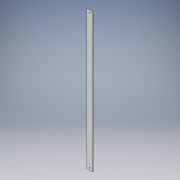
# Autodesk Inventor part: Strutural Integrity Bar
Saved by Autodesk Inventor 2018 (Build 220112000, 112)
## iProperties
Created: 2019-01-10
Part Number: Strutural Integrity Bar
Material: Generic
Document SubType Name: Modeling
Designer: maste
Density: 1 g/cm^3
Appearance: Default
Author: maste
Autodesk Inventor part; units mm, degrees
ref_plane "YZ Plane" through (0, 0, 0) normal (1, 0, 0) x (0, 1, 0)
ref_plane "XZ Plane" through (0, 0, 0) normal (0, 1, 0) x (-1, 0, 0)
ref_plane "XY Plane" through (0, 0, 0) normal (0, 0, 1) x (1, 0, 0)
sketch "Sketch1" plane through (0, 0, 0) normal (0, 0, 1) x (1, 0, 0)
  line L0 (0, 0) -> (25.4, 0)
  line L1 (25.4, 0) -> (25.4, 635)
  line L2 (25.4, 635) -> (0, 635)
  line L3 (0, 635) -> (0, 0)
  line L4 (12.7, 0) -> (12.7, 10.3251) construction
  circle A0 centre (12.7, 10.3251) radius 2.5797
  line L5 (12.7, 635) -> (12.7, 624.6749) construction
  circle A1 centre (12.7, 624.6749) radius 2.5797
  dimension "d0" = 25.4
  dimension "d1" = 635
  dimension "d2" = 10.3251
  dimension "d3" = 5.1594
  dimension "d4" = 10.3251
  constraints: 12 end point, 2 centre point, 2 coincident, 2 midpoint, 2 parallel, 2 vertical, 1 horizontal, 1 perpendicular
  measures "d0" distance of L2.end L1.end
  measures "d1" distance of L1.end L0.end
  measures "d2" distance of L4.start L4.end
  measures "d3" diameter of A0
  measures "d4" distance of L5.start L5.end
extrude "Extrusion1" add sketch "Sketch1" along normal blind 3.175
body "Solid1"
